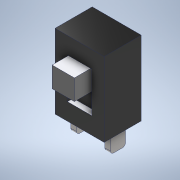
# Autodesk Inventor part: Switch_Base
Saved by Autodesk Inventor 2022 (Build 260153000, 153)
## iProperties
Created: 2022-12-26
Part Number: Switch_Base
Material: Generic
Document SubType Name: Modeling
Designer: karpova
Density: 1 g/cm^3
Appearance: PTFE
Author: karpova
Autodesk Inventor part; units mm, degrees
ref_plane "YZ Plane" through (0, 0, 0) normal (1, 0, 0) x (0, 1, 0)
ref_plane "XZ Plane" through (0, 0, 0) normal (0, 1, 0) x (-1, 0, 0)
ref_plane "XY Plane" through (0, 0, 0) normal (0, 0, 1) x (1, 0, 0)
sketch "Sketch1" plane through (0, 0, 0) normal (0, 0, 1) x (1, 0, 0)
  line L0 (-4.19, 6.35) -> (4.19, 6.35)
  line L1 (4.19, 6.35) -> (4.19, -6.35)
  line L2 (4.19, -6.35) -> (-4.19, -6.35)
  line L3 (-4.19, -6.35) -> (-4.19, 6.35)
  line L4 (0, 0) -> (4.19, 0) construction
  line L5 (0, 0) -> (0, -6.35) construction
  dimension "d0" = 8.38
  dimension "d1" = 12.7
  constraints: 12 end point, 2 horizontal, 2 midpoint, 2 parallel, 1 perpendicular, 1 vertical
  measures "d0" distance between parallel lines of L1 L3
  measures "d1" distance of L0.end L1.end
extrude "Extrusion1" add sketch "Sketch1" along normal blind 6.35
sketch "Sketch2" plane through (0, 0, 6.35) normal (0, 0, 1) x (1, 0, 0)
  line L0 (0, 0) -> (0, 14.132) construction
  line L1 (-2.075, 3.45) -> (2.075, 3.45)
  line L2 (2.075, 3.45) -> (2.075, -3.45)
  line L3 (2.075, -3.45) -> (-2.075, -3.45)
  line L4 (-2.075, -3.45) -> (-2.075, 3.45)
  line L5 (2.075, 0.15) -> (2.075, -3.45)
  line L6 (2.075, -3.45) -> (-2.075, -3.45)
  line L7 (-2.075, -3.45) -> (-2.075, 0.15)
  line L8 (0, 0) -> (4.19, 0) construction
  line L9 (4.19, -6.35) -> (4.19, 6.35) construction
  dimension "d4" = 4.15
  dimension "d20" = 6.9
  constraints: 18 end point, 3 parallel, 1 horizontal, 1 midpoint, 1 perpendicular, 1 point on line, 1 vertical, 2 other
  measures "d4" distance between parallel lines of L2 L4
  measures "d20" distance between parallel lines of L3 L1
extrude "Extrusion2" cut sketch "Sketch2" against normal blind 1
sketch "Sketch3" plane through (0, 0, 6.35) normal (0, 0, 1) x (1, 0, 0)
  line L0 (0, 0) -> (0, 14.132) construction
  line L1 (-1.905, 3.45) -> (1.905, 3.45)
  line L2 (1.905, 3.45) -> (1.905, -3.45)
  line L3 (1.905, -3.45) -> (-1.905, -3.45)
  line L4 (-1.905, -3.45) -> (-1.905, 3.45)
  line L5 (-1.905, -0.06) -> (1.905, -0.06)
  line L6 (1.905, -0.06) -> (1.905, -3.45)
  line L7 (1.905, -3.45) -> (-1.905, -3.45)
  line L8 (-1.905, -3.45) -> (-1.905, -0.06)
  line L9 (0, 0) -> (4.19, 0) construction
  line L10 (4.19, -6.35) -> (4.19, 6.35) construction
  line L11 (-2.075, 3.45) -> (2.075, 3.45) projected
  line L12 (2.075, -3.45) -> (-2.075, -3.45) projected
  point P0 (1.905, -0.06)
  dimension "d9" = 3.81
  dimension "d11" = 3.51
  constraints: 22 end point, 4 parallel, 2 collinear, 2 horizontal, 2 perpendicular, 1 midpoint, 1 point on line, 1 vertical, 2 other
  measures "d9" distance between parallel lines of L2 L4
  measures "d11" distance between parallel lines of L5 L1
extrude "Extrusion3" add sketch "Sketch3" along normal blind 9.14 from surface at -6.35 contours L1 L2 L5 L4
sketch "Sketch4" plane through (-4.19, -6.35, 0) normal (0, -1, 0) x (1, 0, 0)
  line L0 (0, 0) -> (0, 6.35) construction
  line L1 (0, 3.175) -> (8.38, 3.175) construction
  line L2 (8.38, 0) -> (8.38, 6.35) construction
  line L3 (4.19, 0) -> (4.19, 6.35) construction
  line L4 (8.38, 6.35) -> (0, 6.35) construction
  line L5 (6.6, 4.445) -> (7.59, 4.445)
  line L6 (7.59, 4.445) -> (7.59, 1.905)
  line L7 (7.59, 1.905) -> (6.6, 1.905)
  line L8 (6.6, 1.905) -> (6.6, 4.445)
  line L9 (7.095, 4.445) -> (7.095, 1.905) construction
  line L10 (1.78, 4.445) -> (0.79, 4.445)
  line L11 (0.79, 4.445) -> (0.79, 1.905)
  line L12 (0.79, 1.905) -> (1.78, 1.905)
  line L13 (1.78, 1.905) -> (1.78, 4.445)
  line L14 (1.285, 4.445) -> (1.285, 1.905) construction
  dimension "d14" = 0.99
  dimension "d15" = 2.54
  dimension "d24" = 6.8
  constraints: 24 end point, 6 symmetric about line, 5 midpoint, 2 parallel, 1 horizontal, 1 perpendicular, 1 other
  measures "d14" distance between parallel lines of L6 L8
  measures "d15" distance between parallel lines of L7 L5
  measures "d24" distance between parallel lines of L11 L6
extrude "Extrusion4" add sketch "Sketch4" along normal blind 3.16
fillet "Fillet1" radius 0.51 4 edges at (-2.905, -9.51, 4.445) (-2.905, -9.51, 1.905) (2.905, -9.51, 4.445) (2.905, -9.51, 1.905)
equation "\"d7\" = switchTrackExtrusion"
equation "\"switchTrackExtrusion\" = 1"
body "Solid1"
